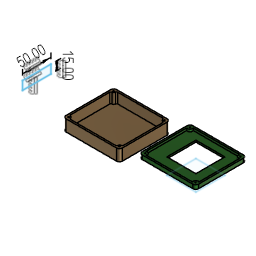
PCB+Box+V1 (Autodesk Fusion 360 design; units mm, degrees)
Autodesk Fusion 360 part; units mm, degrees
sketch "Sketch5" plane through (0, 0, 0) normal (0, 0, 1) x (1, 0, 0)
  line L0 (78, 79) -> (-1, 79)
  line L1 (-8, 72) -> (-8, 3)
  line L2 (-1, -4) -> (78, -4)
  line L3 (85, 3) -> (85, 72)
  line L4 (0, 75) -> (65, 75)
  line L5 (0, 0) -> (0, 75)
  line L6 (65, 0) -> (0, 0)
  line L7 (65, 75) -> (65, 0)
  line L8 (-11, 77) -> (-11, -2)
  arc A0 (-11, -2) -> (-6, -7) centre (-6, -2) ccw
  line L9 (-6, -7) -> (83, -7)
  arc A1 (83, -7) -> (88, -2) centre (83, -2) ccw
  line L10 (88, -2) -> (88, 77)
  arc A2 (88, 77) -> (83, 82) centre (83, 77) ccw
  line L11 (83, 82) -> (-6, 82)
  arc A3 (-6, 82) -> (-11, 77) centre (-6, 77) ccw
  circle A4 centre (-6, -2) radius 1.45
  arc A5 (-3, -2) -> (-6, 1) centre (-6, -2) ccw
  arc A6 (-8, 3) -> (-6, 1) centre (-6, 3) ccw
  arc A7 (-3, -2) -> (-1, -4) centre (-1, -2) ccw
  circle A8 centre (-6, 77) radius 1.45
  arc A9 (-6, 74) -> (-3, 77) centre (-6, 77) ccw
  arc A10 (-6, 74) -> (-8, 72) centre (-6, 72) ccw
  arc A11 (-1, 79) -> (-3, 77) centre (-1, 77) ccw
  circle A12 centre (83, 77) radius 1.45
  arc A13 (80, 77) -> (83, 74) centre (83, 77) ccw
  arc A14 (80, 77) -> (78, 79) centre (78, 77) ccw
  arc A15 (85, 72) -> (83, 74) centre (83, 72) ccw
  circle A16 centre (83, -2) radius 1.45
  arc A17 (83, 1) -> (80, -2) centre (83, -2) ccw
  arc A18 (78, -4) -> (80, -2) centre (78, -2) ccw
  arc A19 (83, 1) -> (85, 3) centre (83, 3) ccw
  line L12 (0, 0) -> (65, 0)
  line L13 (65, 0) -> (65, 75)
  line L14 (65, 75) -> (0, 75)
  line L15 (0, 75) -> (0, 0)
  circle A20 centre (-6, 77) radius 1.125
  circle A21 centre (83, 77) radius 1.125
  circle A22 centre (83, -2) radius 1.125
  circle A23 centre (-6, -2) radius 1.125
  dimension "d29" = 4
  dimension "d30" = 8
  dimension "d31" = 4
  dimension "d32" = 20
  dimension "d35" = 2.9
  dimension "d36" = 6
  dimension "d37" = 2
  dimension "d38" = 2
  dimension "d39" = 2.9
  dimension "d40" = 6
  dimension "d41" = 2
  dimension "d42" = 2.9
  dimension "d43" = 6
  dimension "d44" = 2
  dimension "d45" = 2.9
  dimension "d46" = 6
  dimension "d47" = 2
  dimension "d55" = 2.25
  dimension "d56" = 2.25
  dimension "d57" = 2.25
  dimension "d58" = 2.25
  constraint horizontal L0
  constraint vertical L1
  constraint horizontal L2
  constraint vertical L3
  constraint concentric A4 A5
  constraint tangent A2 L11
  constraint tangent L10 A2
  constraint tangent L8 A3
  constraint tangent L9 A1
  constraint tangent A0 L9
  constraint tangent L8 A0
  constraint tangent A1 L10
  constraint tangent L11 A3
  constraint tangent L1 A6
  constraint tangent A5 A6
  constraint tangent A5 A7
  constraint tangent L2 A7
  constraint concentric A3 A8
  constraint concentric A8 A9
  constraint tangent L1 A10
  constraint tangent A9 A10
  constraint tangent A9 A11
  constraint tangent L0 A11
  constraint equal A10 A11
  constraint concentric A2 A13
  constraint tangent L0 A14
  constraint tangent A13 A14
  constraint tangent L3 A15
  constraint tangent A13 A15
  constraint equal A14 A15
  constraint concentric A1 A16
  constraint concentric A16 A17
  constraint tangent L2 A18
  constraint tangent A17 A18
  constraint tangent L3 A19
  constraint tangent A17 A19
  constraint equal A18 A19
  constraint horizontal L12
  constraint vertical L13
  constraint horizontal L14
  constraint vertical L15
  constraint coincident L4.end L7.start
  constraint coincident L5.start L6.end
  constraint concentric A9 A20
  constraint concentric A12 A21
  constraint concentric A17 A22
  constraint concentric A5 A23
  measures "d29" distance of L0 L4
  measures "d30" distance of L1 L5
  measures "d31" distance of L2 L6
  measures "d32" distance of L3 L7
  measures "d35" diameter of A4
  measures "d36" diameter of A5
  measures "d37" radius of A6
  measures "d38" radius of A7
  measures "d39" diameter of A8
  measures "d40" diameter of A9
  measures "d41" radius of A10
  measures "d42" diameter of A12
  measures "d43" diameter of A13
  measures "d44" radius of A14
  measures "d45" diameter of A16
  measures "d46" diameter of A17
  measures "d47" radius of A18
  measures "d55" diameter of A20
  measures "d56" diameter of A21
  measures "d57" diameter of A22
  measures "d58" diameter of A23
extrude "Extrude1" add sketch "Sketch5" along normal blind 2 contours L0 L1 L2 L3 A5 A6 A7 A9 A10 A11 A13 A14 A15 A17 A18 A19 | L4 L5 L6 L7 L12 L13 L14 L15 makes body 1
extrude "Extrude2" add sketch "Sketch5" along normal blind 20 separate body contours L8 A0 L9 A1 L10 A2 L11 A3 | A4 | A8 | A12 | A16 | A20 | A21 | A22 | A23 makes body 2
extrude "Extrude3" cut sketch "Sketch5" along normal blind 20 from surface at 4 contours A4 | A8 | A12 | A16 | A20 | A21 | A22 | A23 bodies 2
extrude "Extrude4" add sketch "Sketch5" along normal blind 7 from surface at 25 separate body contours L0 L1 L2 L3 A5 A6 A7 A9 A10 A11 A13 A14 A15 A17 A18 A19 | L4 L5 L6 L7 L12 L13 L14 L15 | L8 A0 L9 A1 L10 A2 L11 A3 | A4 | A8 | A12 | A16 makes body 3
move_body "Move2" bodies 3 to x (1, 0, 0) y (0, 1, 0) z (0, 0, 1) at (134, 0, 0)
shell "Shell1" thickness 3 removed faces 1 at (157.9839, 50.3939, 32) on bodies 3
sketch "Sketch7" plane through (0, 0, 0) normal (0, 0, 1) x (1, 0, 0)
  line L0 (148.7399, 66.6637) -> (199.7399, 66.6637)
  line L1 (199.7399, 66.6637) -> (199.7399, 15.6637)
  line L2 (199.7399, 15.6637) -> (148.7399, 15.6637)
  line L3 (148.7399, 15.6637) -> (148.7399, 66.6637)
  dimension "d63" = 51
  dimension "d64" = 51
  constraint horizontal L0
  constraint vertical L1
  constraint horizontal L2
  constraint vertical L3
  measures "d63" distance of L0.start L0.end
  measures "d64" distance of L0.start L2.end
extrude "Extrude5" cut sketch "Sketch7" along normal blind 31 bodies 3
sketch "Sketch8" plane through (0, 0, 0) normal (1, 0, 0) x (0, 1, 0)
  line L0 (65.5289, 17.5249, -104.9096) -> (15.5289, 17.5249, -104.9096)
  line L1 (15.5289, 17.5249, -104.9096) -> (15.5289, 2.5249, -104.9096)
  line L2 (15.5289, 2.5249, -104.9096) -> (65.5289, 2.5249, -104.9096)
  line L3 (65.5289, 2.5249, -104.9096) -> (65.5289, 17.5249, -104.9096)
  dimension "d67" = 50
  dimension "d68" = 15
extrude "Extrude6" [rolled back] along distance 100 taper angle 0
sketch "New Box" plane through (0, 0, 0) normal (0, 0, 1) x (1, 0, 0)
  line L0 (-41.403, 25) -> (61.487, 25)
  line L1 (61.487, 25) -> (61.487, -27.44)
  line L2 (61.487, -27.44) -> (-41.403, -27.44)
  line L3 (-41.403, -27.44) -> (-41.403, 25)
  dimension "d71" = 102.89
  dimension "d72" = 52.44
  dimension "d73" = -8
  constraint horizontal L0
  constraint vertical L1
  constraint horizontal L2
  constraint vertical L3
  measures "d71" distance of L0.start L0.end
  measures "d72" distance of L0.start L2.end
named bodies: "BOX_BOTTOM", "BOX_SIDES", "BOX_LID"
